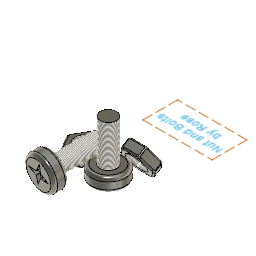
Nuts and Bolts v3 (Autodesk Fusion 360 design; units mm, degrees)
Autodesk Fusion 360 part; units mm, degrees
sketch "Sketch1" plane through (0, 0, 0) normal (0, 0, 1) x (1, 0, 0)
  circle A0 centre (0, 0) radius 25
  constraint coincident A0.centre origin
extrude "Extrude1" add sketch "Sketch1" along normal blind 20 makes body 1
sketch "Sketch2" plane through (0, 0, 20) normal (0, 0, 1) x (-1, 0, 0)
  circle A0 centre (0, 0) radius 25
  circle A1 centre (0, 0) radius 12.7605
  constraint coincident A0.centre A1.centre
extrude "Extrude2" add sketch "Sketch2" along normal blind 60 contours A1 bodies 1
thread "Thread1" "ISO Metric profile 26.0 M26x1.5 6g" major diameter 25.85 minor diameter 24.1319 pitch 1.5 angle 60 resizes the face on face at (-12.6971, 1.2705, 60) on bodies 1
fillet "Fillet1" radius 5 1 faces at (24.9689, 1.2461, 6.6667) on bodies 1
sketch "Sketch3" plane through (0, 0, 0) normal (0, 0, -1) x (1, 0, 0)
  circle A0 centre (0, 0) radius 20
  line L0 (0.3477, 17.161) -> (-2.6124, 3.3157)
  line L1 (0.3477, 17.161) -> (2.9627, 3.6188)
  line L2 (4.2249, -3.3217) -> (16.1969, -1.0099)
  line L3 (16.1969, -1.0099) -> (2.9627, 3.6188)
  line L4 (4.2249, -3.3217) -> (-0.201, -15.9758)
  line L5 (-0.201, -15.9758) -> (-2.592, -3.5931)
  circle A1 through (12.925, 0, -80) (-6.4625, 11.1934, -80) (-6.4625, -11.1934, -80)
  line L6 (-2.6124, 3.3157) -> (-13.8658, 0.3014)
  line L7 (-13.8658, 0.3014) -> (-2.592, -3.5931)
  constraint perpendicular L1 L2
  constraint perpendicular L3 L4
  constraint perpendicular L2 L5
extrude "Extrude3" cut sketch "Sketch3" against normal blind 5 contours L0 L1 L2 L3 L4 L5 L6 L7 bodies 1
thread "Thread2" "ISO Metric profile 25.0 M25x2 6g" major diameter 24.822 minor diameter 22.5289 pitch 2 angle 60 resizes the face on face at (-12.8608, -1.2869, 40) on bodies 1
sketch "Sketch4" plane through (0, 0, 0) normal (0, 0, 1) x (1, 0, 0)
  line L0 (0, 75) -> (-12.5, 53.3494)
  line L1 (-12.5, 53.3494) -> (0, 31.6987)
  line L2 (0, 31.6987) -> (25, 31.6987)
  line L3 (25, 31.6987) -> (37.5, 53.3494)
  line L4 (37.5, 53.3494) -> (25, 75)
  line L5 (25, 75) -> (0, 75)
  point P0 (12.5, 53.3494)
extrude "Extrude4" add sketch "Sketch4" along normal blind 15 separate body makes body 2
hole "Hole1" at (12.4304, 54.1256, 15) direction (0, 0, -1) diameter 30 depth 15 tip angle 180 bodies 2
thread "Thread3" "ISO Metric profile 33.0 M33x3.5 6H" major diameter 33.3925 minor diameter 29.4911 pitch 3.5 angle 60 resizes the face on face at (13.9239, 39.2001, 10) on bodies 2
fillet "Fillet2" radius 2 6 faces at (-8.3333, 46.1325, 5) (-4.1667, 67.7831, 5) (8.3333, 31.6987, 5) (33.3333, 46.1325, 10) (16.6667, 75, 5) (33.3333, 60.5662, 5) on bodies 2
thread "Thread4" "ISO Metric profile 24.0 M24x3 6g" major diameter 23.7645 minor diameter 20.3295 pitch 3 angle 60 resizes the face on face at (-12.3493, -1.2357, 40) on bodies 1
sketch "Sketch5" plane through (0, 0, 0) normal (0, 0, 1) x (1, 0, 0)
copy_body "CopyPasteBodies1" bodies 1 makes body 3
move_body "Move1" bodies 3 to x (1, 0, 0) y (0, 1, 0) z (0, 0, 1) at (-33.7206, -47.7608, 2.0013)
copy_body "CopyPasteBodies2" bodies 2 makes body 4
move_body "Move2" bodies 4 to x (1, 0, 0) y (0, 1, 0) z (0, 0, 1) at (-60, -40, 0)
move_body "Move3" bodies 3 to x (0.087156, 0.086824, 0.992404) y (0.98106, 0.165507, -0.100639) z (-0.172987, 0.982379, -0.070755) at (18.0389, -57.6729, 52.1025)
move_body "Move4" bodies 3 to x (0.999886, 0.00065, -0.015115) y (0.00065, 0.996309, 0.085835) z (0.015115, -0.085835, 0.996195) at (-0.3924, 2.2282, 10.9892)
move_body "Move5" bodies 3 to x (0.999385, -0.014925, -0.031746) y (0.020109, 0.985269, 0.169827) z (0.028743, -0.170361, 0.984962) at (0.0686, 3.7772, 7.1876)
move_body "Move6" bodies 3 to x (1, 0, 0) y (0, 1, 0) z (0, 0, 1) at (0.1147, 0.3992, -1.9564)
move_body "Move7" bodies 3 to x (0.966038, -0.252788, -0.053567) y (0.253567, 0.967283, 0.008185) z (0.049745, -0.02149, 0.998531) at (13.7139, -12.3785, -1.7219)
move_body "Move8" bodies 2 to x (1, 0, 0) y (0, 1, 0) z (0, 0, 1) at (5, 8.6603, 0)
move_body "Move9" bodies 3 to x (0.999934, -0.000598, -0.011484) y (-0.000598, 0.994588, -0.103896) z (0.011484, 0.103896, 0.994522) at (-0.316, -2.8587, -6.794)
sketch "Sketch6" plane through (0, 0, 0) normal (0, 0, 1) x (1, 0, 0)
move_body "Move10" bodies 2 to x (1, 0, 0) y (0, -0.5, 0.866025) z (0, -0.866025, -0.5) at (0, 67.7622, -28.4271)
sketch "Sketch7" plane through (0, 0, 0) normal (0, 0, 1) x (1, 0, 0)
  line L0 (50, 150) -> (-50, 150) construction
  line L1 (-50, 150) -> (-50, 100) construction
  line L2 (-50, 100) -> (50, 100) construction
  line L3 (50, 100) -> (50, 150) construction
  dimension "d24" = 10
